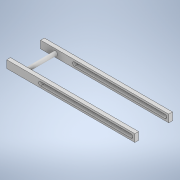
# Autodesk Inventor part: Base
Saved by Autodesk Inventor 2021 (Build 250183000, 183)
## iProperties
Created: 2021-04-01
Part Number: Base
Material: Generic
Document SubType Name: Modeling
Designer: Darek
Density: 1 g/cm^3
Appearance: Default
Author: Darek
Autodesk Inventor part; units mm, degrees
ref_plane "YZ Plane" through (0, 0, 0) normal (1, 0, 0) x (0, 1, 0)
ref_plane "XZ Plane" through (0, 0, 0) normal (0, 1, 0) x (-1, 0, 0)
ref_plane "XY Plane" through (0, 0, 0) normal (0, 0, 1) x (1, 0, 0)
sketch "Sketch1" plane through (0, 0, 0) normal (0, 0, 1) x (1, 0, 0)
  point P0 (0, 0)
sketch "Sketch2" plane through (0, 0, 0) normal (0, 0, 1) x (1, 0, 0)
  line L0 (0, 0) -> (170, 0)
  line L1 (170, 0) -> (170, 10)
  line L2 (170, 10) -> (0, 10)
  line L3 (0, 10) -> (0, 0)
  circle A0 centre (165, 5) radius 2.5
  circle A1 centre (45, 5) radius 2.5
  line L4 (45, 2.5) -> (165, 2.5)
  line L5 (165, 2.5) -> (165, 7.5)
  line L6 (165, 7.5) -> (45, 7.5)
  line L7 (45, 7.5) -> (45, 2.5)
  point P0 (45, 7.5)
  point P1 (165, 2.5)
  dimension "d4" = 5
  dimension "d5" = 5
  dimension "d0" = 170
  dimension "d1" = 10
  dimension "d2" = 5
  dimension "d3" = 5
  dimension "d6" = 120
  dimension "d7" = 5
  dimension "d8" = 2.5
  dimension "d9" = 2.5
  constraints: 16 end point, 3 perpendicular, 2 horizontal, 2 parallel, 1 vertical, 6 other
  measures "d0" distance between parallel lines of L1 L3
  measures "d1" distance between parallel lines of L0 L2
  measures "d2" distance from line of point (165, 5) L1
  measures "d3" distance from line of point (165, 5) L2
  measures "d6" distance of point (45, 5) point (165, 5)
  measures "d7" distance from line of L0 point (45, 5)
  measures "d8" distance between parallel lines of L0 L4
  measures "d9" distance between parallel lines of L2 L6
extrude "Extrusion1" add sketch "Sketch2" along normal blind 50
sketch "Sketch3" plane through (0, 10, 0) normal (0, 1, 0) x (1, 0, 0)
  line L0 (170, 0) -> (170, -50) projected
  line L1 (170, -45) -> (-20, -45)
  line L2 (-20, -45) -> (-20, -5)
  line L3 (-20, -5) -> (170, -5)
  line L4 (170, -5) -> (170, -45)
  line L5 (170, -50) -> (0, -50) projected
  line L6 (170, 0) -> (0, 0) projected
  dimension "d12" = 190
  dimension "d13" = 5
  dimension "d14" = 5
  constraints: 8 end point, 2 parallel, 1 horizontal, 1 perpendicular, 1 point on line
  measures "d12" distance between parallel lines of L0 L2
  measures "d13" distance between parallel lines of L5 L1
  measures "d14" distance between parallel lines of L6 L3
extrude "Extrusion2" cut sketch "Sketch3" against normal blind 10
sketch "Sketch4" plane through (0, 0, 0) normal (0, 0, -1) x (-1, 0, 0)
  circle A0 centre (-20, 5) radius 2.5
  line L0 (0, 10) -> (0, 0) projected
  line L1 (0, 0) -> (-170, 0) projected
  dimension "d17" = 20
  dimension "d18" = 5
  dimension "d19" = 5
  constraints: 1 centre point
  measures "d17" distance from line of L0 A0.centre
  measures "d18" diameter of A0
  measures "d19" distance from line of L1 A0.centre
extrude "Extrusion3" add sketch "Sketch4" along normal blind 1 and the other way blind 50
body "Solid1"
